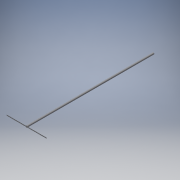
# Autodesk Inventor part: Long Rod
Saved by Autodesk Inventor 2017.2 (Build 212233000, 233)
## iProperties
Created: 2017-03-31
Part Number: Long Rod
Material: Generic
Document SubType Name: Modeling
Designer: haden
Density: 1 g/cm^3
Appearance: Default
Author: haden
Autodesk Inventor part; units mm, degrees
ref_plane "YZ Plane" through (0, 0, 0) normal (1, 0, 0) x (0, 1, 0)
ref_plane "XZ Plane" through (0, 0, 0) normal (0, 1, 0) x (-1, 0, 0)
ref_plane "XY Plane" through (0, 0, 0) normal (0, 0, 1) x (1, 0, 0)
sketch "Sketch1" plane through (0, 0, 0) normal (0, 0, 1) x (1, 0, 0)
  circle A0 centre (0, 0) radius 2500
  dimension "d0" = 5000
  constraints: 1 centre point, 1 coincident
  measures "d0" diameter of A0
extrude "Extrusion1" add sketch "Sketch1" along normal blind 350000
sketch "Sketch2" plane through (0, 0, 350000) normal (0, 0, 1) x (1, 0, 0)
  line L0 (-55000, 1250) -> (55000, 1250)
  line L1 (55000, 1250) -> (55000, -1250)
  line L2 (55000, -1250) -> (-55000, -1250)
  line L3 (-55000, -1250) -> (-55000, 1250)
  circle A0 centre (0, 0) radius 2500 projected
  point P0 (0, 1250)
  dimension "d3" = 110000
  dimension "d4" = 2500
  dimension "d5" = 1250
  constraints: 8 end point, 2 parallel, 1 horizontal, 1 midpoint, 1 perpendicular, 1 vertical alignment
  measures "d3" distance of L0.start L0.end
  measures "d4" distance of L2.end L0.start
  measures "d5" distance from line of L0 point (0, 0)
extrude "Extrusion2" add sketch "Sketch2" along normal blind 100 contours L0 A0 L2 L3 | L0 A0 L2 | L0 L1 L2 A0
body "Solid1"
